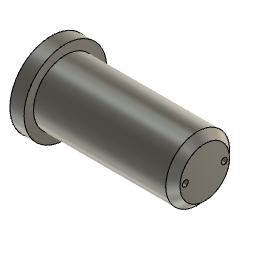
DesignExercise (Autodesk Fusion 360 design; units mm, degrees)
Autodesk Fusion 360 part; units mm, degrees
sketch "Sketch1" plane through (0, 0, 0) normal (1, 0, 0) x (0, 1, 0)
  circle A0 centre (0, 0) radius 2.7
  constraint coincident A0.centre origin
extrude "Extrude1" add sketch "Sketch1" along normal blind 13
sketch "Sketch2" plane through (0, 0, 0) normal (1, 0, 0) x (0, 1, 0)
  circle A0 centre (0, 0) radius 3.5
  constraint coincident A0.centre origin
extrude "Extrude2" add sketch "Sketch2" along normal blind 1.2
chamfer "Chamfer1" distance 0.6 angle 45 1 edges at (13, -2.5173, -0.9764)
hole "Hole1" at (0, 0, 0) direction (1, 0, 0) diameter 4.2 depth 5 tip angle 180
sketch "Sketch3" plane through (5, 0, 0) normal (-1, 0, 0) x (0, -1, 0)
  circle A0 centre (0, 0) radius 2.1
  line L0 (0, 0) -> (-1.9, 0)
  line L1 (0, 0) -> (1.9, 0)
  line L2 (0, 0.4) -> (0, -0.25)
  circle A1 centre (1.65, 0) radius 0.25
  circle A2 centre (-1.65, 0) radius 0.25
  constraint coincident A0.centre L0.start
  constraint horizontal L0
  constraint parallel L0 L1
  constraint vertical L2
  constraint coincident L1 A1.centre
  constraint coincident L1.end A1
  constraint symmetric L2 A1 A2
hole "Hole2" at (5, -1.65, 0) at (5, 1.65, 0) direction (1, 0, 0) diameter 0.5 end through all
